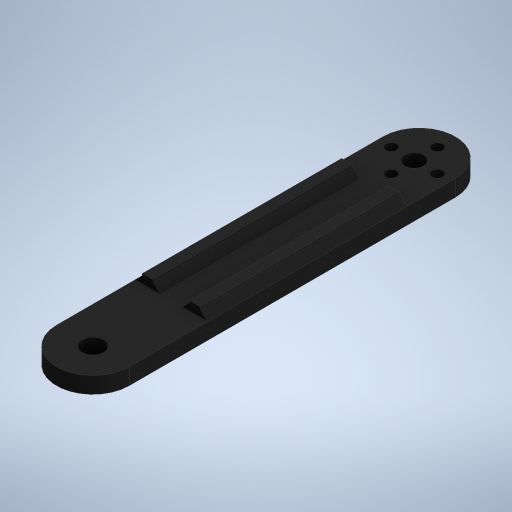
# Autodesk Inventor part: link1_print_v2
Saved by Autodesk Inventor 2023 (Build 270158000, 158)
## iProperties
Created: 2023-11-03
Part Number: link1_print_v2
Material: Ogólny
Document SubType Name: Modeling
Designer: janek
Density: 1 g/cm^3
Appearance: Domyślna
Author: janek
## iProperties of the stored document link1_print_Drukowanie 3D.ipt
Created: 2023-11-13
Part Number: link1_print_Drukowanie 3D
Material: Ogólny
Document SubType Name: Modeling
Designer: janek
Density: 1 g/cm^3
Appearance: Domyślna
Author: janek
Autodesk Inventor part; units mm, degrees
ref_plane "YZ Plane" through (0, 0, 0) normal (1, 0, 0) x (0, 1, 0)
ref_plane "XZ Plane" through (0, 0, 0) normal (0, 1, 0) x (-1, 0, 0)
ref_plane "XY Plane" through (0, 0, 0) normal (0, 0, 1) x (1, 0, 0)
sketch "Szkic1" plane through (0, 0, 0) normal (0, 1, 0) x (-1, 0, 0)
  line L0 (10, 55) -> (-10, 55)
  line L1 (-10, 55) -> (-10, -55)
  line L2 (-10, -55) -> (10, -55)
  line L3 (10, -55) -> (10, 55)
  line L4 (10, 55) -> (-10, -55) construction
  line L5 (-10, 55) -> (10, -55) construction
  circle A0 centre (0, -43.65) radius 2.6
  circle A1 centre (0, -37.3) radius 1.5
  circle A2 centre (0, -50) radius 1.5
  circle A3 centre (-6.35, -43.65) radius 1.5
  circle A4 centre (6.35, -43.65) radius 1.5
  line L6 (6.35, -43.65) -> (-6.35, -43.65)
  line L7 (0, -37.3) -> (0, -50)
  point P0 (0, 0)
  dimension "d0" = 20
  dimension "d1" = 110
  dimension "d2" = 5.2
  dimension "d3" = 3
  dimension "d4" = 3
  dimension "d5" = 6.35
  dimension "d6" = 6.35
  dimension "d7" = 5
  dimension "d22" = 3
  dimension "d23" = 3
  dimension "d24" = 6.35
  dimension "d25" = 6.35
  dimension "d26" = 8.9803
  dimension "d27" = 8.9803
  dimension "d28" = 3.65
  constraints: 16 end point, 5 centre point, 2 horizontal, 2 midpoint, 2 parallel, 1 perpendicular, 1 vertical
  measures "d0" distance of L2.end L1.end
  measures "d1" distance between parallel lines of L2 L0
  measures "d2" diameter of A0
  measures "d3" diameter of A1
  measures "d4" diameter of A2
  measures "d5" distance of L7.start A0.centre
  measures "d6" distance of L7.end A0.centre
  measures "d7" distance from line of L2 L7.end
  measures "d22" diameter of A3
  measures "d23" diameter of A4
  measures "d24" distance of A0.centre L6.start
  measures "d25" distance of A0.centre L6.end
  measures "d26" distance of L6.end L7.start
  measures "d27" distance of L7.end L6.end
  measures "d28" distance from line of L3 L6.start
extrude "Wyciągnięcie proste1" add sketch "Szkic1" along normal blind 4.5 contours L3 L2 L1 L0 | A3 | A4
sketch "Szkic3" plane through (0, 4.5, 0) normal (0, 1, 0) x (1, 0, 0)
  circle A0 centre (0, -45) radius 2.5 projected
  circle A1 centre (0, -45) radius 2.5
  point P0 (0, 0)
  constraints: 1 centre point, 1 coincident
fillet "Zaokrąglenie1" radius 10 4 edges at (10, 2.25, -55) (-10, 2.25, -55) (10, 2.25, 55) (-10, 2.25, 55)
extrude "Wyciągnięcie proste4" cut sketch "Szkic3" against normal blind 10
sketch "Szkic4" plane through (0, 4.5, 0) normal (0, 1, 0) x (1, 0, 0)
  circle A0 centre (0, -45) radius 2.5 projected
  circle A1 centre (0, -45) radius 3
  point P0 (0, 0)
  dimension "d19" = 6
  constraints: 1 centre point, 1 coincident
  measures "d19" diameter of A1
extrude "Wyciągnięcie proste5" cut sketch "Szkic4" against normal blind 10
extrude "Wyciągnięcie proste6" cut sketch "Szkic1" along normal blind 7 contours A3 | A4
sketch "Szkic5" plane through (0, 4.5, 0) normal (0, 1, 0) x (1, 0, 0)
  line L0 (-8, -23.35) -> (-5, -23.35)
  line L1 (-5, -23.35) -> (-5, 31.65)
  line L2 (-5, 31.65) -> (-8, 31.65)
  line L3 (-8, 31.65) -> (-8, -23.35)
  line L4 (5, -23.35) -> (8, -23.35)
  line L5 (8, -23.35) -> (8, 31.65)
  line L6 (8, 31.65) -> (5, 31.65)
  line L7 (5, 31.65) -> (5, -23.35)
  circle A0 centre (0, 43.65) radius 2.6 projected
  line L8 (10, -45) -> (10, 45) projected
  line L9 (-10, 45) -> (-10, -45) projected
  point P0 (0, 0)
  point P1 (6.5, 31.65)
  point P2 (6.5, -23.35)
  point P3 (-6.5, 31.65)
  point P4 (-6.5, -23.35)
  dimension "d31" = 55
  dimension "d32" = 55
  dimension "d33" = 67
  dimension "d34" = 3
  dimension "d35" = 3
  dimension "d36" = 2
  dimension "d37" = 2
  constraints: 16 end point, 4 midpoint, 4 parallel, 2 horizontal, 2 perpendicular, 1 point on line
  measures "d31" distance of point (6.5, 31.65) point (6.5, -23.35)
  measures "d32" distance of point (-6.5, 31.65) point (-6.5, -23.35)
  measures "d33" vertical distance of point (-6.5, -23.35) A0.centre
  measures "d34" distance between parallel lines of L3 L1
  measures "d35" distance between parallel lines of L7 L5
  measures "d36" distance between parallel lines of L5 L8
  measures "d37" distance between parallel lines of L9 L3
extrude "Wyciągnięcie proste7" add sketch "Szkic5" along normal blind 2.5 contours L3 L2 L1 L0 | L7 L6 L5 L4
chamfer "Faza1" distance 2 angle 45 4 edges at (8, 4.5, -4.15) (-5, 4.5, -4.15) (-8, 4.5, -4.15) (5, 4.5, -4.15)
